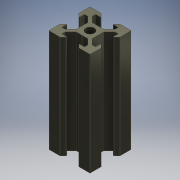
# Autodesk Inventor part: Vslot_2020
Saved by Autodesk Inventor 2016 (Build 200138000, 138)
## iProperties
Created: 2021-06-30
Part Number: Vslot_2020
Material: Generic
Document SubType Name: Modeling
Designer: TG
Density: 1 g/cm^3
Appearance: Gunmetal
Author: TG
Autodesk Inventor part; units mm, degrees
ref_plane "YZ Plane" through (0, 0, 0) normal (1, 0, 0) x (0, 1, 0)
ref_plane "XZ Plane" through (0, 0, 0) normal (0, 1, 0) x (-1, 0, 0)
ref_plane "XY Plane" through (0, 0, 0) normal (0, 0, 1) x (1, 0, 0)
sketch "Sketch1" plane through (0, 0, 0) normal (0, 0, 1) x (1, 0, 0)
  line L0 (-3.2054, 8.7057) -> (-4.6311, 10.1314)
  arc A0 (-4.6311, 10.1314) -> (-4.7018, 10.1607) centre (-4.7018, 10.0607) ccw
  line L1 (-4.7018, 10.1607) -> (-9.8804, 10.1607)
  arc A1 (-9.8804, 10.1607) -> (-10.0804, 9.9607) centre (-9.8804, 9.9607) ccw
  line L2 (-10.0804, 9.9607) -> (-10.0804, 4.7821)
  arc A2 (-10.0804, 4.7821) -> (-10.0511, 4.7114) centre (-9.9804, 4.7821) ccw
  line L3 (-10.0511, 4.7114) -> (-8.6254, 3.2857)
  line L4 (-3.2054, 8.3607) -> (-5.5804, 8.3607)
  arc A3 (-0.0804, 2.2607) -> (-1.5653, 1.6456) centre (-0.0804, 0.1607) ccw
  line L5 (-5.5804, 8.3607) -> (-5.5804, 6.7628)
  arc A4 (-5.5804, 6.7628) -> (-5.5511, 6.6921) centre (-5.4804, 6.7628) ccw
  line L6 (-5.5511, 6.6921) -> (-2.949, 4.09)
  arc A5 (-2.949, 4.09) -> (-2.8783, 4.0607) centre (-2.8783, 4.1607) ccw
  line L7 (-2.8783, 4.0607) -> (-0.2142, 4.0607)
  line L8 (-3.2054, 8.7057) -> (-3.2054, 8.3607)
  line L9 (3.0446, 8.7057) -> (4.4703, 10.1314)
  arc A6 (4.5411, 10.1607) -> (4.4703, 10.1314) centre (4.5411, 10.0607) ccw
  line L10 (4.5411, 10.1607) -> (9.7196, 10.1607)
  arc A7 (9.9196, 9.9607) -> (9.7196, 10.1607) centre (9.7196, 9.9607) ccw
  line L11 (9.9196, 9.9607) -> (9.9196, 4.7821)
  arc A8 (9.8903, 4.7114) -> (9.9196, 4.7821) centre (9.8196, 4.7821) ccw
  line L12 (9.8903, 4.7114) -> (8.4646, 3.2857)
  line L13 (3.0446, 8.3607) -> (5.4196, 8.3607)
  arc A9 (1.4046, 1.6456) -> (-0.0804, 2.2607) centre (-0.0804, 0.1607) ccw
  line L14 (5.4196, 8.3607) -> (5.4196, 6.7628)
  arc A10 (5.3903, 6.6921) -> (5.4196, 6.7628) centre (5.3196, 6.7628) ccw
  line L15 (5.3903, 6.6921) -> (2.7883, 4.09)
  arc A11 (2.7176, 4.0607) -> (2.7883, 4.09) centre (2.7176, 4.1607) ccw
  line L16 (2.7176, 4.0607) -> (0.0535, 4.0607)
  line L17 (3.0446, 8.7057) -> (3.0446, 8.3607)
  line L18 (-0.2142, 4.0607) -> (-0.0804, 3.9562)
  line L19 (0.0535, 4.0607) -> (-0.0804, 3.9562)
  line L20 (8.1196, 3.2857) -> (8.1196, 5.6607)
  arc A12 (2.0196, 0.1607) -> (1.4046, 1.6456) centre (-0.0804, 0.1607) ccw
  line L21 (8.1196, 5.6607) -> (6.5217, 5.6607)
  arc A13 (6.5217, 5.6607) -> (6.451, 5.6314) centre (6.5217, 5.5607) ccw
  line L22 (6.451, 5.6314) -> (3.8489, 3.0293)
  arc A14 (3.8489, 3.0293) -> (3.8196, 2.9586) centre (3.9196, 2.9586) ccw
  line L23 (3.8196, 2.9586) -> (3.8196, 0.2946)
  line L24 (8.4646, 3.2857) -> (8.1196, 3.2857)
  line L25 (-8.2804, 3.2857) -> (-8.2804, 5.6607)
  arc A15 (-1.5653, 1.6456) -> (-2.1804, 0.1607) centre (-0.0804, 0.1607) ccw
  line L26 (-8.2804, 5.6607) -> (-6.6824, 5.6607)
  arc A16 (-6.6117, 5.6314) -> (-6.6824, 5.6607) centre (-6.6824, 5.5607) ccw
  line L27 (-6.6117, 5.6314) -> (-4.0097, 3.0293)
  arc A17 (-3.9804, 2.9586) -> (-4.0097, 3.0293) centre (-4.0804, 2.9586) ccw
  line L28 (-3.9804, 2.9586) -> (-3.9804, 0.2946)
  line L29 (-8.6254, 3.2857) -> (-8.2804, 3.2857)
  line L30 (-3.2054, -8.3843) -> (-4.6311, -9.81)
  arc A18 (-4.7018, -9.8393) -> (-4.6311, -9.81) centre (-4.7018, -9.7393) ccw
  line L31 (-4.7018, -9.8393) -> (-9.8804, -9.8393)
  arc A19 (-10.0804, -9.6393) -> (-9.8804, -9.8393) centre (-9.8804, -9.6393) ccw
  line L32 (-10.0804, -9.6393) -> (-10.0804, -4.4607)
  arc A20 (-10.0511, -4.39) -> (-10.0804, -4.4607) centre (-9.9804, -4.4607) ccw
  line L33 (-10.0511, -4.39) -> (-8.6254, -2.9643)
  line L34 (-3.2054, -8.0393) -> (-5.5804, -8.0393)
  arc A21 (-1.5653, -1.3242) -> (-0.0804, -1.9393) centre (-0.0804, 0.1607) ccw
  line L35 (-5.5804, -8.0393) -> (-5.5804, -6.4414)
  arc A22 (-5.5511, -6.3707) -> (-5.5804, -6.4414) centre (-5.4804, -6.4414) ccw
  line L36 (-5.5511, -6.3707) -> (-2.949, -3.7686)
  arc A23 (-2.8783, -3.7393) -> (-2.949, -3.7686) centre (-2.8783, -3.8393) ccw
  line L37 (-2.8783, -3.7393) -> (-0.2142, -3.7393)
  line L38 (-3.2054, -8.3843) -> (-3.2054, -8.0393)
  line L39 (3.0446, -8.0393) -> (5.4196, -8.0393)
  arc A24 (-0.0804, -1.9393) -> (1.4046, -1.3242) centre (-0.0804, 0.1607) ccw
  line L40 (5.4196, -8.0393) -> (5.4196, -6.4414)
  arc A25 (5.4196, -6.4414) -> (5.3903, -6.3707) centre (5.3196, -6.4414) ccw
  line L41 (5.3903, -6.3707) -> (2.7883, -3.7686)
  arc A26 (2.7883, -3.7686) -> (2.7176, -3.7393) centre (2.7176, -3.8393) ccw
  line L42 (2.7176, -3.7393) -> (0.0535, -3.7393)
  line L43 (3.0446, -8.3843) -> (3.0446, -8.0393)
  line L44 (-0.2142, -3.7393) -> (-0.0804, -3.6348)
  line L45 (0.0535, -3.7393) -> (-0.0804, -3.6348)
  line L46 (8.4646, -2.9643) -> (9.8903, -4.39)
  arc A27 (9.9196, -4.4607) -> (9.8903, -4.39) centre (9.8196, -4.4607) ccw
  line L47 (9.9196, -4.4607) -> (9.9196, -9.6393)
  arc A28 (9.7196, -9.8393) -> (9.9196, -9.6393) centre (9.7196, -9.6393) ccw
  line L48 (9.7196, -9.8393) -> (4.5411, -9.8393)
  arc A29 (4.4703, -9.81) -> (4.5411, -9.8393) centre (4.5411, -9.7393) ccw
  line L49 (4.4703, -9.81) -> (3.0446, -8.3843)
  line L50 (8.1196, -2.9643) -> (8.1196, -5.3393)
  arc A30 (1.4046, -1.3242) -> (2.0196, 0.1607) centre (-0.0804, 0.1607) ccw
  line L51 (8.1196, -5.3393) -> (6.5217, -5.3393)
  arc A31 (6.451, -5.31) -> (6.5217, -5.3393) centre (6.5217, -5.2393) ccw
  line L52 (6.451, -5.31) -> (3.8489, -2.7079)
  arc A32 (3.8196, -2.6372) -> (3.8489, -2.7079) centre (3.9196, -2.6372) ccw
  line L53 (3.8196, -2.6372) -> (3.8196, 0.0269)
  line L54 (8.4646, -2.9643) -> (8.1196, -2.9643)
  line L55 (-8.2804, -2.9643) -> (-8.2804, -5.3393)
  arc A33 (-2.1804, 0.1607) -> (-1.5653, -1.3242) centre (-0.0804, 0.1607) ccw
  line L56 (-8.2804, -5.3393) -> (-6.6824, -5.3393)
  arc A34 (-6.6824, -5.3393) -> (-6.6117, -5.31) centre (-6.6824, -5.2393) ccw
  line L57 (-6.6117, -5.31) -> (-4.0097, -2.7079)
  arc A35 (-4.0097, -2.7079) -> (-3.9804, -2.6372) centre (-4.0804, -2.6372) ccw
  line L58 (-3.9804, -2.6372) -> (-3.9804, 0.0269)
  line L59 (-8.6254, -2.9643) -> (-8.2804, -2.9643)
  line L60 (-3.9804, 0.0269) -> (-3.8759, 0.1607)
  line L61 (-3.9804, 0.2946) -> (-3.8759, 0.1607)
  line L62 (0.0535, -3.7393) -> (-0.0804, -3.6348)
  line L63 (-0.2142, -3.7393) -> (-0.0804, -3.6348)
  line L64 (3.8196, 0.2946) -> (3.7152, 0.1607)
  line L65 (3.8196, 0.0269) -> (3.7152, 0.1607)
  point P0 (0, 0)
  constraints: 132 end point, 72 point on circle, 36 centre point
extrude "Extrusion1" add sketch "Sketch1" along normal blind 50
body "Solid1"
